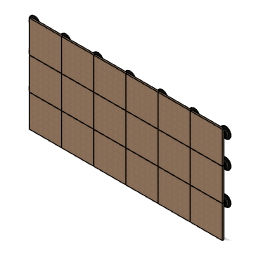
Balkon (Autodesk Fusion 360 archive; units mm, degrees)
design "Balkon2"
Autodesk Fusion 360 part; units mm, degrees
sketch "Skizze1" plane through (0, 0, 0) normal (0, 0, 1) x (1, 0, 0)
  line L0 (-1895, 890) -> (1895, 890)
  line L1 (1895, 890) -> (1895, -890)
  line L2 (1895, -890) -> (-1895, -890)
  line L3 (-1895, -890) -> (-1895, 890)
  line L4 (-1895, 890) -> (1895, -890) construction
  line L5 (1895, 890) -> (-1895, -890) construction
  line L6 (-1895, -490) -> (-1495, -890)
  line L7 (-1895, -490) -> (-1305.4449, -490) construction
  line L8 (1895, -490) -> (1495, -890)
  dimension "d1" = 1780
  dimension "d2" = 3790
  dimension "d3" = 45
  dimension "d4" = 400
  dimension "d5" = 45
  constraint horizontal L0
  constraint perpendicular L0 L1
  constraint parallel L0 L2
  constraint parallel L1 L3
  constraint coincident L4 origin
  constraint coincident L5 origin
  constraint horizontal L7
  constraint coincident L3 L6.start
  constraint coincident L1 L8.start
  constraint coincident L2 L8.end
  constraint coincident L2 L6.end
  constraint horizontal L6.start L8.start
  measures "d1" distance of L0.start L2.end
  measures "d2" distance of L0.start L0.end
  measures "d3" angle of L6 L7
  measures "d4" distance of L2 L8.start
  measures "d5" angle of L2 L8
sketch "Skizze2" plane through (0, 0, 10) normal (0, 0, 1) x (1, 0, 0)
  line L0 (-1895, -490) -> (-1495, -890)
  line L1 (-1495, -890) -> (1495, -890)
  line L2 (1495, -890) -> (1895, -490)
  line L3 (1895, -490) -> (1895, 890)
  line L4 (1895, 890) -> (-1895, 890)
  line L5 (-1895, 890) -> (-1895, -490)
  line L6 (-1995, 990) -> (1995, 990)
  line L7 (1995, 990) -> (1995, 890)
  line L8 (1995, 890) -> (-1995, 890)
  line L9 (-1995, 890) -> (-1995, 990)
  line L10 (1995, 890) -> (1895, 890)
  line L11 (1895, 890) -> (1895, -490)
  line L12 (1895, -490) -> (1995, -490)
  line L13 (1995, -490) -> (1995, 890)
  line L14 (-1995, 890) -> (-1895, 890)
  line L15 (-1895, 890) -> (-1895, -490)
  line L16 (-1895, -490) -> (-1995, -490)
  line L17 (-1995, -490) -> (-1995, 890)
  line L18 (-1995, -490) -> (-1595, -890)
  line L19 (-1595, -890) -> (-1495, -890)
  line L20 (1995, -490) -> (1595, -890)
  line L21 (1595, -890) -> (1495, -890)
  dimension "d8" = 100
  constraint horizontal L6
  constraint vertical L7
  constraint horizontal L8
  constraint vertical L9
  constraint horizontal L10
  constraint vertical L11
  constraint horizontal L12
  constraint vertical L13
  constraint coincident L2.end L3.start
  constraint horizontal L14
  constraint vertical L15
  constraint horizontal L16
  constraint vertical L17
  constraint coincident L0.start L5.end
  constraint coincident L0.end L1.start
  constraint parallel L1 L19
  constraint coincident L1.end L2.start
  constraint parallel L1 L21
  constraint parallel L2 L20
  constraint parallel L0 L18
  constraint equal L9 L14
  constraint equal L10 L14
  constraint collinear L4 L8
  measures "d8" distance of L6.start L8.end
sketch "Skizze1 (2)" plane through (0, 0, 10) normal (0, 0, 1) x (1, 0, 0) in component "Terassenlager"
  line L0 (-1895, -490) -> (-1495, -890)
  line L1 (-1495, -890) -> (1495, -890)
  line L2 (1495, -890) -> (1895, -490)
  line L3 (1895, -490) -> (1895, 890)
  line L4 (1895, 890) -> (-1895, 890)
  line L5 (-1895, 890) -> (-1895, -490)
  circle A0 centre (0, 0) radius 100
  dimension "d13" = 200
  constraint coincident A0.centre origin
  measures "d13" diameter of A0
extrude "Extrusion1" add sketch "Skizze1 (2)" along normal blind 5 contours A0 makes body 1 in component "Terassenlager"
sketch "Skizze2 (2)" plane through (0, 0, 15) normal (0, 0, 1) x (1, 0, 0) in component "Terassenlager"
  circle A0 centre (0, 0) radius 100
  circle A1 centre (0, 0) radius 60
  dimension "d16" = 120
  constraint concentric A0 A1
  measures "d16" diameter of A1
extrude "Extrusion2" add sketch "Skizze2 (2)" along normal blind 40 contours A1 bodies 1 in component "Terassenlager"
sketch "Skizze3" plane through (0, 0, 55) normal (0, 0, 1) x (1, 0, 0) in component "Terassenlager"
  circle A0 centre (0, 0) radius 60
  circle A1 centre (0, 0) radius 40
  line L0 (-1.5, 40) -> (1.5, 40)
  line L1 (1.5, 40) -> (1.5, -40)
  line L2 (1.5, -40) -> (-1.5, -40)
  line L3 (-1.5, -40) -> (-1.5, 40)
  line L4 (-1.5, 40) -> (1.5, -40) construction
  line L5 (1.5, 40) -> (-1.5, -40) construction
  line L6 (40, 1.5) -> (-40, 1.5)
  line L7 (-40, 1.5) -> (-40, -1.5)
  line L8 (-40, -1.5) -> (40, -1.5)
  line L9 (40, -1.5) -> (40, 1.5)
  line L10 (40, 1.5) -> (-40, -1.5) construction
  line L11 (-40, 1.5) -> (40, -1.5) construction
  dimension "d19" = 80
  dimension "d20" = 3
  dimension "d21" = 80
  constraint coincident A0.centre A1.centre
  constraint horizontal L0
  constraint perpendicular L0 L1
  constraint parallel L0 L2
  constraint parallel L1 L3
  constraint coincident L4 A0.centre
  constraint coincident L5 A0.centre
  constraint horizontal L6
  constraint perpendicular L6 L7
  constraint parallel L6 L8
  constraint parallel L7 L9
  constraint coincident L10 A0.centre
  constraint coincident L11 A0.centre
  constraint equal L2 L9
  constraint equal L1 L6
  measures "d19" diameter of A1
  measures "d20" distance of L1.end L2.end
  measures "d21" distance of L0.end L1.end
extrude "Extrusion3" add sketch "Skizze3" along normal blind 3 contours A1 L1 L6 | A1 L1 L8 | A1 L3 L6 | A1 L3 L8 bodies 1 in component "Terassenlager"
sketch "Skizze1 (3)" plane through (0, 0, 0) normal (0, 0, 1) x (1, 0, 0) in component "Platte6060"
  line L0 (0, 0) -> (-600, 0)
  line L1 (-600, 0) -> (-600, -600)
  line L2 (-600, -600) -> (0, -600)
  line L3 (0, -600) -> (0, 0)
  dimension "d60" = 600
  dimension "d61" = 600
  constraint horizontal L0
  constraint vertical L1
  constraint horizontal L2
  constraint vertical L3
  constraint coincident L0.start L3.end
  measures "d60" distance of L0.start L0.end
  measures "d61" distance of L0.start L2.end
extrude "Extrusion1'" add sketch "Skizze1 (3)" along normal blind 30 separate body makes body 2 in component "Platte6060"
pattern_linear "弁25" [suppressed]
pattern_linear "码2" [suppressed]
component "Terassenlager" placed x (1, 0, 0) y (0, 1, 0) z (0, 0, 1) at (1.5, 278.5, 0)
component "Platte6060" placed x (1, 0, 0) y (0, 1, 0) z (0, 0, 1) at (0, 880, 60)
component "Platte6060" placed x (1, 0, 0) y (0, 1, 0) z (0, 0, 1) at (-1206, 880, 60)
component "Platte6060" placed x (1, 0, 0) y (0, 1, 0) z (0, 0, 1) at (-603, 880, 60)
component "Platte6060" placed x (1, 0, 0) y (0, 1, 0) z (0, 0, 1) at (603, 880, 60)
component "Platte6060" placed x (1, 0, 0) y (0, 1, 0) z (0, 0, 1) at (1206, 880, 60)
component "Platte6060" placed x (1, 0, 0) y (0, 1, 0) z (0, 0, 1) at (1809, 880, 60)
component "Platte6060" placed x (1, 0, 0) y (0, 1, 0) z (0, 0, 1) at (-1206, 277, 60)
component "Platte6060" placed x (1, 0, 0) y (0, 1, 0) z (0, 0, 1) at (-603, 277, 60)
component "Platte6060" placed x (1, 0, 0) y (0, 1, 0) z (0, 0, 1) at (0, 277, 60)
component "Platte6060" placed x (1, 0, 0) y (0, 1, 0) z (0, 0, 1) at (603, 277, 60)
component "Platte6060" placed x (1, 0, 0) y (0, 1, 0) z (0, 0, 1) at (1206, 277, 60)
component "Platte6060" placed x (1, 0, 0) y (0, 1, 0) z (0, 0, 1) at (1809, 277, 60)
component "Platte6060" placed x (1, 0, 0) y (0, 1, 0) z (0, 0, 1) at (-1206, -326, 60)
component "Platte6060" placed x (1, 0, 0) y (0, 1, 0) z (0, 0, 1) at (-603, -326, 60)
component "Platte6060" placed x (1, 0, 0) y (0, 1, 0) z (0, 0, 1) at (0, -326, 60)
component "Platte6060" placed x (1, 0, 0) y (0, 1, 0) z (0, 0, 1) at (603, -326, 60)
component "Platte6060" placed x (1, 0, 0) y (0, 1, 0) z (0, 0, 1) at (1206, -326, 60)
component "Platte6060" placed x (1, 0, 0) y (0, 1, 0) z (0, 0, 1) at (1809, -326, 60)
component "Terassenlager" placed x (1, 0, 0) y (0, 1, 0) z (0, 0, 1) at (-1807.5, 881.5, 0)
component "Terassenlager" placed x (1, 0, 0) y (0, 1, 0) z (0, 0, 1) at (-1807.5, 278.5, 0)
component "Terassenlager" placed x (1, 0, 0) y (0, 1, 0) z (0, 0, 1) at (-1807.5, -324.5, 0)
component "Terassenlager" placed x (1, 0, 0) y (0, 1, 0) z (0, 0, 1) at (-1807.5, -927.5, 0)
component "Terassenlager" placed x (1, 0, 0) y (0, 1, 0) z (0, 0, 1) at (-1204.5, 881.5, 0)
component "Terassenlager" placed x (1, 0, 0) y (0, 1, 0) z (0, 0, 1) at (-1204.5, 278.5, 0)
component "Terassenlager" placed x (1, 0, 0) y (0, 1, 0) z (0, 0, 1) at (-1204.5, -324.5, 0)
component "Terassenlager" placed x (1, 0, 0) y (0, 1, 0) z (0, 0, 1) at (-1204.5, -927.5, 0)
component "Terassenlager" placed x (1, 0, 0) y (0, 1, 0) z (0, 0, 1) at (-601.5, 881.5, 0)
component "Terassenlager" placed x (1, 0, 0) y (0, 1, 0) z (0, 0, 1) at (-601.5, 278.5, 0)
component "Terassenlager" placed x (1, 0, 0) y (0, 1, 0) z (0, 0, 1) at (-601.5, -324.5, 0)
component "Terassenlager" placed x (1, 0, 0) y (0, 1, 0) z (0, 0, 1) at (-601.5, -927.5, 0)
component "Terassenlager" placed x (1, 0, 0) y (0, 1, 0) z (0, 0, 1) at (1.5, 881.5, 0)
component "Terassenlager" placed x (1, 0, 0) y (0, 1, 0) z (0, 0, 1) at (1.5, -324.5, 0)
component "Terassenlager" placed x (1, 0, 0) y (0, 1, 0) z (0, 0, 1) at (1.5, -927.5, 0)
component "Terassenlager" placed x (1, 0, 0) y (0, 1, 0) z (0, 0, 1) at (604.5, 881.5, 0)
component "Terassenlager" placed x (1, 0, 0) y (0, 1, 0) z (0, 0, 1) at (604.5, 278.5, 0)
component "Terassenlager" placed x (1, 0, 0) y (0, 1, 0) z (0, 0, 1) at (604.5, -324.5, 0)
component "Terassenlager" placed x (1, 0, 0) y (0, 1, 0) z (0, 0, 1) at (604.5, -927.5, 0)
component "Terassenlager" placed x (1, 0, 0) y (0, 1, 0) z (0, 0, 1) at (1207.5, 881.5, 0)
component "Terassenlager" placed x (1, 0, 0) y (0, 1, 0) z (0, 0, 1) at (1207.5, 278.5, 0)
component "Terassenlager" placed x (1, 0, 0) y (0, 1, 0) z (0, 0, 1) at (1207.5, -324.5, 0)
component "Terassenlager" placed x (1, 0, 0) y (0, 1, 0) z (0, 0, 1) at (1207.5, -927.5, 0)
component "Terassenlager" placed x (1, 0, 0) y (0, 1, 0) z (0, 0, 1) at (1810.5, 881.5, 0)
component "Terassenlager" placed x (1, 0, 0) y (0, 1, 0) z (0, 0, 1) at (1810.5, 278.5, 0)
component "Terassenlager" placed x (1, 0, 0) y (0, 1, 0) z (0, 0, 1) at (1810.5, -324.5, 0)
component "Terassenlager" placed x (1, 0, 0) y (0, 1, 0) z (0, 0, 1) at (1810.5, -927.5, 0)
equation "d5 = d3"

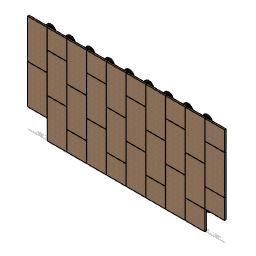
design "Balkon1"
Autodesk Fusion 360 part; units mm, degrees
sketch "Skizze1" plane through (0, 0, 0) normal (0, 0, 1) x (1, 0, 0)
  line L0 (-1895, 890) -> (1895, 890)
  line L1 (1895, 890) -> (1895, -890)
  line L2 (1895, -890) -> (-1895, -890)
  line L3 (-1895, -890) -> (-1895, 890)
  line L4 (-1895, 890) -> (1895, -890) construction
  line L5 (1895, 890) -> (-1895, -890) construction
  line L6 (-1895, -490) -> (-1495, -890)
  line L7 (-1895, -490) -> (-1305.4449, -490) construction
  line L8 (1895, -490) -> (1495, -890)
  dimension "d1" = 1780
  dimension "d2" = 3790
  dimension "d3" = 45
  dimension "d4" = 400
  dimension "d5" = 45
  constraint horizontal L0
  constraint perpendicular L0 L1
  constraint parallel L0 L2
  constraint parallel L1 L3
  constraint coincident L4 origin
  constraint coincident L5 origin
  constraint horizontal L7
  constraint coincident L3 L6.start
  constraint coincident L1 L8.start
  constraint coincident L2 L8.end
  constraint coincident L2 L6.end
  constraint horizontal L6.start L8.start
  measures "d1" distance of L0.start L2.end
  measures "d2" distance of L0.start L0.end
  measures "d3" angle of L6 L7
  measures "d4" distance of L2 L8.start
  measures "d5" angle of L2 L8
sketch "Skizze2" plane through (0, 0, 10) normal (0, 0, 1) x (1, 0, 0)
  line L0 (-1895, -490) -> (-1495, -890)
  line L1 (-1495, -890) -> (1495, -890)
  line L2 (1495, -890) -> (1895, -490)
  line L3 (1895, -490) -> (1895, 890)
  line L4 (1895, 890) -> (-1895, 890)
  line L5 (-1895, 890) -> (-1895, -490)
  line L6 (-1995, 990) -> (1995, 990)
  line L7 (1995, 990) -> (1995, 890)
  line L8 (1995, 890) -> (-1995, 890)
  line L9 (-1995, 890) -> (-1995, 990)
  line L10 (1995, 890) -> (1895, 890)
  line L11 (1895, 890) -> (1895, -490)
  line L12 (1895, -490) -> (1995, -490)
  line L13 (1995, -490) -> (1995, 890)
  line L14 (-1995, 890) -> (-1895, 890)
  line L15 (-1895, 890) -> (-1895, -490)
  line L16 (-1895, -490) -> (-1995, -490)
  line L17 (-1995, -490) -> (-1995, 890)
  line L18 (-1995, -490) -> (-1595, -890)
  line L19 (-1595, -890) -> (-1495, -890)
  line L20 (1995, -490) -> (1595, -890)
  line L21 (1595, -890) -> (1495, -890)
  dimension "d8" = 100
  constraint horizontal L6
  constraint vertical L7
  constraint horizontal L8
  constraint vertical L9
  constraint horizontal L10
  constraint vertical L11
  constraint horizontal L12
  constraint vertical L13
  constraint coincident L2.end L3.start
  constraint horizontal L14
  constraint vertical L15
  constraint horizontal L16
  constraint vertical L17
  constraint coincident L0.start L5.end
  constraint coincident L0.end L1.start
  constraint parallel L1 L19
  constraint coincident L1.end L2.start
  constraint parallel L1 L21
  constraint parallel L2 L20
  constraint parallel L0 L18
  constraint equal L9 L14
  constraint equal L10 L14
  constraint collinear L4 L8
  measures "d8" distance of L6.start L8.end
sketch "Skizze1 (2)" plane through (0, 0, 10) normal (0, 0, 1) x (1, 0, 0) in component "Terassenlager"
  line L0 (-1895, -490) -> (-1495, -890)
  line L1 (-1495, -890) -> (1495, -890)
  line L2 (1495, -890) -> (1895, -490)
  line L3 (1895, -490) -> (1895, 890)
  line L4 (1895, 890) -> (-1895, 890)
  line L5 (-1895, 890) -> (-1895, -490)
  circle A0 centre (0, 0) radius 100
  dimension "d13" = 200
  constraint coincident A0.centre origin
  measures "d13" diameter of A0
extrude "Extrusion1" add sketch "Skizze1 (2)" along normal blind 5 contours A0 makes body 1 in component "Terassenlager"
sketch "Skizze2 (2)" plane through (0, 0, 15) normal (0, 0, 1) x (1, 0, 0) in component "Terassenlager"
  circle A0 centre (0, 0) radius 100
  circle A1 centre (0, 0) radius 60
  dimension "d16" = 120
  constraint concentric A0 A1
  measures "d16" diameter of A1
extrude "Extrusion2" add sketch "Skizze2 (2)" along normal blind 40 contours A1 bodies 1 in component "Terassenlager"
sketch "Skizze3" plane through (0, 0, 55) normal (0, 0, 1) x (1, 0, 0) in component "Terassenlager"
  circle A0 centre (0, 0) radius 60
  circle A1 centre (0, 0) radius 40
  line L0 (-1.5, 40) -> (1.5, 40)
  line L1 (1.5, 40) -> (1.5, -40)
  line L2 (1.5, -40) -> (-1.5, -40)
  line L3 (-1.5, -40) -> (-1.5, 40)
  line L4 (-1.5, 40) -> (1.5, -40) construction
  line L5 (1.5, 40) -> (-1.5, -40) construction
  line L6 (40, 1.5) -> (-40, 1.5)
  line L7 (-40, 1.5) -> (-40, -1.5)
  line L8 (-40, -1.5) -> (40, -1.5)
  line L9 (40, -1.5) -> (40, 1.5)
  line L10 (40, 1.5) -> (-40, -1.5) construction
  line L11 (-40, 1.5) -> (40, -1.5) construction
  dimension "d19" = 80
  dimension "d20" = 3
  dimension "d21" = 80
  constraint coincident A0.centre A1.centre
  constraint horizontal L0
  constraint perpendicular L0 L1
  constraint parallel L0 L2
  constraint parallel L1 L3
  constraint coincident L4 A0.centre
  constraint coincident L5 A0.centre
  constraint horizontal L6
  constraint perpendicular L6 L7
  constraint parallel L6 L8
  constraint parallel L7 L9
  constraint coincident L10 A0.centre
  constraint coincident L11 A0.centre
  constraint equal L2 L9
  constraint equal L1 L6
  measures "d19" diameter of A1
  measures "d20" distance of L1.end L2.end
  measures "d21" distance of L0.end L1.end
extrude "Extrusion3" add sketch "Skizze3" along normal blind 3 contours A1 L1 L6 | A1 L1 L8 | A1 L3 L6 | A1 L3 L8 bodies 1 in component "Terassenlager"
sketch "Skizze1 (3)" plane through (0, 0, 0) normal (0, 0, 1) x (1, 0, 0) in component "PLatte4080"
  line L0 (0, 0) -> (-400, 0)
  line L1 (-400, 0) -> (-400, -800)
  line L2 (-400, -800) -> (0, -800)
  line L3 (0, -800) -> (0, 0)
  dimension "d32" = 400
  dimension "d33" = 800
  constraint horizontal L0
  constraint vertical L1
  constraint horizontal L2
  constraint vertical L3
  constraint coincident L0.start L3.end
  measures "d32" distance of L0.start L0.end
  measures "d33" distance of L0.start L2.end
extrude "Extrusion1'" add sketch "Skizze1 (3)" along normal blind 30 separate body makes body 2 in component "PLatte4080"
sketch "Skizze1 (4)" plane through (0, 0, 0) normal (0, 0, 1) x (1, 0, 0) in component "Platte4040"
  line L0 (0, 0) -> (-400, 0)
  line L1 (-400, 0) -> (-400, -400)
  line L2 (-400, -400) -> (0, -400)
  line L3 (0, -400) -> (0, 0)
  dimension "d36" = 400
  dimension "d37" = 400
  constraint horizontal L0
  constraint vertical L1
  constraint horizontal L2
  constraint vertical L3
  constraint coincident L0.start L3.end
  measures "d36" distance of L0.start L0.end
  measures "d37" distance of L0.start L2.end
extrude "Extrusion1''" add sketch "Skizze1 (4)" along normal blind 30 separate body makes body 3 in component "Platte4040"
pattern_linear "堁14" [suppressed]
pattern_linear "堁\u000e\u0000\u0000\u0000Ā໸\u0000\u0000\u0000\u0000" [suppressed]
pattern_linear "14" [suppressed]
pattern_linear "ⴁ17" [suppressed]
form "Form1" [no effect]
pattern_linear "码2" [suppressed]
component "Terassenlager" placed x (1, 0, 0) y (0, 1, 0) z (0, 0, 1) at (-2010.8981, 78.0969, 0)
component "PLatte4080" placed x (1, 0, 0) y (0, 1, 0) z (0, 0, 1) at (0, 880, 60)
component "Platte4040" placed x (1, 0, 0) y (0, 1, 0) z (0, 0, 1) at (403, 880, 60)
component "PLatte4080" placed x (1, 0, 0) y (0, 1, 0) z (0, 0, 1) at (-1612, 880, 60)
component "PLatte4080" placed x (1, 0, 0) y (0, 1, 0) z (0, 0, 1) at (-1209, 477, 60)
component "PLatte4080" placed x (1, 0, 0) y (0, 1, 0) z (0, 0, 1) at (-806, 880, 60)
component "PLatte4080" placed x (1, 0, 0) y (0, 1, 0) z (0, 0, 1) at (-403, 477, 60)
component "PLatte4080" placed x (1, 0, 0) y (0, 1, 0) z (0, 0, 1) at (403, 477, 60)
component "PLatte4080" placed x (1, 0, 0) y (0, 1, 0) z (0, 0, 1) at (806, 880, 60)
component "PLatte4080" placed x (1, 0, 0) y (0, 1, 0) z (0, 0, 1) at (1209, 477, 60)
component "PLatte4080" placed x (1, 0, 0) y (0, 1, 0) z (0, 0, 1) at (1612, 880, 60)
component "PLatte4080" placed x (1, 0, 0) y (0, 1, 0) z (0, 0, 1) at (2015, 477, 60)
component "PLatte4080" placed x (1, 0, 0) y (0, 1, 0) z (0, 0, 1) at (0, 77, 60)
component "Platte4040" placed x (1, 0, 0) y (0, 1, 0) z (0, 0, 1) at (1612, -726, 60)
component "PLatte4080" placed x (1, 0, 0) y (0, 1, 0) z (0, 0, 1) at (-1612, 77, 60)
component "PLatte4080" placed x (1, 0, 0) y (0, 1, 0) z (0, 0, 1) at (-1209, -326, 60)
component "PLatte4080" placed x (1, 0, 0) y (0, 1, 0) z (0, 0, 1) at (-806, 77, 60)
component "PLatte4080" placed x (1, 0, 0) y (0, 1, 0) z (0, 0, 1) at (-403, -326, 60)
component "PLatte4080" placed x (1, 0, 0) y (0, 1, 0) z (0, 0, 1) at (403, -326, 60)
component "PLatte4080" placed x (1, 0, 0) y (0, 1, 0) z (0, 0, 1) at (806, 77, 60)
component "PLatte4080" placed x (1, 0, 0) y (0, 1, 0) z (0, 0, 1) at (1209, -326, 60)
component "PLatte4080" placed x (1, 0, 0) y (0, 1, 0) z (0, 0, 1) at (1612, 77, 60)
component "PLatte4080" placed x (1, 0, 0) y (0, 1, 0) z (0, 0, 1) at (2015, -326, 60)
component "Platte4040" placed x (1, 0, 0) y (0, 1, 0) z (0, 0, 1) at (2015, 880, 60)
component "Platte4040" placed x (1, 0, 0) y (0, 1, 0) z (0, 0, 1) at (1209, 880, 60)
component "Platte4040" placed x (1, 0, 0) y (0, 1, 0) z (0, 0, 1) at (-403, 880, 60)
component "Platte4040" placed x (1, 0, 0) y (0, 1, 0) z (0, 0, 1) at (-1209, 880, 60)
component "Platte4040" placed x (1, 0, 0) y (0, 1, 0) z (0, 0, 1) at (806, -726, 60)
component "Platte4040" placed x (1, 0, 0) y (0, 1, 0) z (0, 0, 1) at (0, -726, 60)
component "Platte4040" placed x (1, 0, 0) y (0, 1, 0) z (0, 0, 1) at (-806, -726, 60)
component "Platte4040" placed x (1, 0, 0) y (0, 1, 0) z (0, 0, 1) at (2015, -324, 60)
component "Terassenlager" placed x (1, 0, 0) y (0, 1, 0) z (0, 0, 1) at (-2010.8981, 878.0969, 0)
component "Terassenlager" placed x (1, 0, 0) y (0, 1, 0) z (0, 0, 1) at (-2010.8981, 478.0969, 0)
component "Terassenlager" placed x (1, 0, 0) y (0, 1, 0) z (0, 0, 1) at (-2010.8981, -321.9031, 0)
component "Terassenlager" placed x (1, 0, 0) y (0, 1, 0) z (0, 0, 1) at (-2010.8981, -721.9031, 0)
component "Terassenlager" placed x (1, 0, 0) y (0, 1, 0) z (0, 0, 1) at (-2010.8981, -1121.9031, 0)
component "Terassenlager" placed x (1, 0, 0) y (0, 1, 0) z (0, 0, 1) at (-1610.8981, 878.0969, 0)
component "Terassenlager" placed x (1, 0, 0) y (0, 1, 0) z (0, 0, 1) at (-1610.8981, 478.0969, 0)
component "Terassenlager" placed x (1, 0, 0) y (0, 1, 0) z (0, 0, 1) at (-1610.8981, 78.0969, 0)
component "Terassenlager" placed x (1, 0, 0) y (0, 1, 0) z (0, 0, 1) at (-1610.8981, -321.9031, 0)
component "Terassenlager" placed x (1, 0, 0) y (0, 1, 0) z (0, 0, 1) at (-1610.8981, -721.9031, 0)
component "Terassenlager" placed x (1, 0, 0) y (0, 1, 0) z (0, 0, 1) at (-1610.8981, -1121.9031, 0)
component "Terassenlager" placed x (1, 0, 0) y (0, 1, 0) z (0, 0, 1) at (-1210.8981, 878.0969, 0)
component "Terassenlager" placed x (1, 0, 0) y (0, 1, 0) z (0, 0, 1) at (-1210.8981, 478.0969, 0)
component "Terassenlager" placed x (1, 0, 0) y (0, 1, 0) z (0, 0, 1) at (-1210.8981, 78.0969, 0)
component "Terassenlager" placed x (1, 0, 0) y (0, 1, 0) z (0, 0, 1) at (-1210.8981, -321.9031, 0)
component "Terassenlager" placed x (1, 0, 0) y (0, 1, 0) z (0, 0, 1) at (-1210.8981, -721.9031, 0)
component "Terassenlager" placed x (1, 0, 0) y (0, 1, 0) z (0, 0, 1) at (-1210.8981, -1121.9031, 0)
component "Terassenlager" placed x (1, 0, 0) y (0, 1, 0) z (0, 0, 1) at (-810.8981, 878.0969, 0)
component "Terassenlager" placed x (1, 0, 0) y (0, 1, 0) z (0, 0, 1) at (-810.8981, 478.0969, 0)
component "Terassenlager" placed x (1, 0, 0) y (0, 1, 0) z (0, 0, 1) at (-810.8981, 78.0969, 0)
component "Terassenlager" placed x (1, 0, 0) y (0, 1, 0) z (0, 0, 1) at (-810.8981, -321.9031, 0)
component "Terassenlager" placed x (1, 0, 0) y (0, 1, 0) z (0, 0, 1) at (-810.8981, -721.9031, 0)
component "Terassenlager" placed x (1, 0, 0) y (0, 1, 0) z (0, 0, 1) at (-810.8981, -1121.9031, 0)
component "Terassenlager" placed x (1, 0, 0) y (0, 1, 0) z (0, 0, 1) at (-410.8981, 878.0969, 0)
component "Terassenlager" placed x (1, 0, 0) y (0, 1, 0) z (0, 0, 1) at (-410.8981, 478.0969, 0)
component "Terassenlager" placed x (1, 0, 0) y (0, 1, 0) z (0, 0, 1) at (-410.8981, 78.0969, 0)
component "Terassenlager" placed x (1, 0, 0) y (0, 1, 0) z (0, 0, 1) at (-410.8981, -321.9031, 0)
component "Terassenlager" placed x (1, 0, 0) y (0, 1, 0) z (0, 0, 1) at (-410.8981, -721.9031, 0)
component "Terassenlager" placed x (1, 0, 0) y (0, 1, 0) z (0, 0, 1) at (-410.8981, -1121.9031, 0)
component "Terassenlager" placed x (1, 0, 0) y (0, 1, 0) z (0, 0, 1) at (-10.8981, 878.0969, 0)
component "Terassenlager" placed x (1, 0, 0) y (0, 1, 0) z (0, 0, 1) at (-10.8981, 478.0969, 0)
component "Terassenlager" placed x (1, 0, 0) y (0, 1, 0) z (0, 0, 1) at (-10.8981, 78.0969, 0)
component "Terassenlager" placed x (1, 0, 0) y (0, 1, 0) z (0, 0, 1) at (-10.8981, -321.9031, 0)
component "Terassenlager" placed x (1, 0, 0) y (0, 1, 0) z (0, 0, 1) at (-10.8981, -721.9031, 0)
component "Terassenlager" placed x (1, 0, 0) y (0, 1, 0) z (0, 0, 1) at (-10.8981, -1121.9031, 0)
component "Terassenlager" placed x (1, 0, 0) y (0, 1, 0) z (0, 0, 1) at (389.1019, 878.0969, 0)
component "Terassenlager" placed x (1, 0, 0) y (0, 1, 0) z (0, 0, 1) at (389.1019, 478.0969, 0)
component "Terassenlager" placed x (1, 0, 0) y (0, 1, 0) z (0, 0, 1) at (389.1019, 78.0969, 0)
component "Terassenlager" placed x (1, 0, 0) y (0, 1, 0) z (0, 0, 1) at (389.1019, -321.9031, 0)
component "Terassenlager" placed x (1, 0, 0) y (0, 1, 0) z (0, 0, 1) at (389.1019, -721.9031, 0)
component "Terassenlager" placed x (1, 0, 0) y (0, 1, 0) z (0, 0, 1) at (389.1019, -1121.9031, 0)
component "Terassenlager" placed x (1, 0, 0) y (0, 1, 0) z (0, 0, 1) at (789.1019, 878.0969, 0)
component "Terassenlager" placed x (1, 0, 0) y (0, 1, 0) z (0, 0, 1) at (789.1019, 478.0969, 0)
component "Terassenlager" placed x (1, 0, 0) y (0, 1, 0) z (0, 0, 1) at (789.1019, 78.0969, 0)
component "Terassenlager" placed x (1, 0, 0) y (0, 1, 0) z (0, 0, 1) at (789.1019, -321.9031, 0)
component "Terassenlager" placed x (1, 0, 0) y (0, 1, 0) z (0, 0, 1) at (789.1019, -721.9031, 0)
component "Terassenlager" placed x (1, 0, 0) y (0, 1, 0) z (0, 0, 1) at (789.1019, -1121.9031, 0)
component "Terassenlager" placed x (1, 0, 0) y (0, 1, 0) z (0, 0, 1) at (1189.1019, 878.0969, 0)
component "Terassenlager" placed x (1, 0, 0) y (0, 1, 0) z (0, 0, 1) at (1189.1019, 478.0969, 0)
component "Terassenlager" placed x (1, 0, 0) y (0, 1, 0) z (0, 0, 1) at (1189.1019, 78.0969, 0)
component "Terassenlager" placed x (1, 0, 0) y (0, 1, 0) z (0, 0, 1) at (1189.1019, -321.9031, 0)
component "Terassenlager" placed x (1, 0, 0) y (0, 1, 0) z (0, 0, 1) at (1189.1019, -721.9031, 0)
component "Terassenlager" placed x (1, 0, 0) y (0, 1, 0) z (0, 0, 1) at (1189.1019, -1121.9031, 0)
component "Terassenlager" placed x (1, 0, 0) y (0, 1, 0) z (0, 0, 1) at (1589.1019, 878.0969, 0)
component "Terassenlager" placed x (1, 0, 0) y (0, 1, 0) z (0, 0, 1) at (1589.1019, 478.0969, 0)
component "Terassenlager" placed x (1, 0, 0) y (0, 1, 0) z (0, 0, 1) at (1589.1019, 78.0969, 0)
component "Terassenlager" placed x (1, 0, 0) y (0, 1, 0) z (0, 0, 1) at (1589.1019, -321.9031, 0)
component "Terassenlager" placed x (1, 0, 0) y (0, 1, 0) z (0, 0, 1) at (1589.1019, -721.9031, 0)
component "Terassenlager" placed x (1, 0, 0) y (0, 1, 0) z (0, 0, 1) at (1589.1019, -1121.9031, 0)
component "Terassenlager" placed x (1, 0, 0) y (0, 1, 0) z (0, 0, 1) at (1989.1019, 878.0969, 0)
component "Terassenlager" placed x (1, 0, 0) y (0, 1, 0) z (0, 0, 1) at (1989.1019, 478.0969, 0)
component "Terassenlager" placed x (1, 0, 0) y (0, 1, 0) z (0, 0, 1) at (1989.1019, 78.0969, 0)
component "Terassenlager" placed x (1, 0, 0) y (0, 1, 0) z (0, 0, 1) at (1989.1019, -321.9031, 0)
component "Terassenlager" placed x (1, 0, 0) y (0, 1, 0) z (0, 0, 1) at (1989.1019, -721.9031, 0)
component "Terassenlager" placed x (1, 0, 0) y (0, 1, 0) z (0, 0, 1) at (1989.1019, -1121.9031, 0)
equation "d5 = d3"
